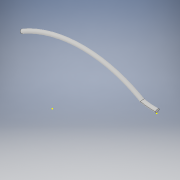
# Autodesk Inventor part: CapBallHolderArmNew
Saved by Autodesk Inventor 2017 (Build 210142000, 142)
## iProperties
Created: 2017-04-24
Part Number: CapBallHolderArmNew
Material: Generic
Document SubType Name: Modeling
Designer: RoboticsUser
Density: 1 g/cm^3
Appearance: Default
Mass: 11.5621 g
Surface Area: 73.9815 cm^2
Volume: 11.5621 cm^3
Author: RoboticsUser
Autodesk Inventor part; units mm, degrees
ref_plane "YZ Plane" through (0, 0, 0) normal (1, 0, 0) x (0, 1, 0)
ref_plane "XZ Plane" through (0, 0, 0) normal (0, 1, 0) x (-1, 0, 0)
ref_plane "XY Plane" through (0, 0, 0) normal (0, 0, 1) x (1, 0, 0)
sketch "Sketch1" plane through (0, 0, 0) normal (0, 0, 1) x (1, 0, 0)
  arc A0 (0, 0) -> (-203.2, 0) centre (-101.6, -175.9764) ccw
  dimension "d0" = 203.2
  dimension "d1" = 203.2
  constraints: 2 point on circle, 1 centre point
  measures "d0" distance of A0.start A0.end
  measures "d1" radius of A0
ref_plane "Work Plane1" through (0, 0, 0) normal (-0.8660254, 0.5, 0) x (-0.5, -0.8660254, 0)
ref_plane "Work Plane2" through (-203.2, 0, 0) normal (-0.8660254, -0.5, 0) x (0.5, -0.8660254, 0)
sketch "Sketch2" plane through (0, 0, 0) normal (-0.8660254, 0.5, 0) x (-0.5, -0.8660254, 0)
  circle A0 centre (0, 0) radius 3.175
  dimension "d2" = 6.35
  constraints: 1 centre point, 1 coincident
  measures "d2" diameter of A0
sketch "Sketch3" plane through (-203.2, 0, 0) normal (-0.8660254, -0.5, 0) x (0.5, -0.8660254, 0)
  circle A0 centre (0, 0) radius 3.175
  point P0 (101.6, 0)
  dimension "d3" = 6.35
  constraints: 1 centre point
  measures "d3" diameter of A0
sweep "Sweep1" add profiles "Sketch3" path "Sketch1"
sketch "Sketch4" plane through (0, 0, 0) normal (-0.8660254, 0.5, 0) x (-0.5, -0.8660254, 0)
  point P0 (0, 0)
sketch "Sketch5" plane through (-203.2, 0, 0) normal (-0.8660254, -0.5, 0) x (0.5, -0.8660254, 0)
  point P0 (101.6, 0)
sketch "Sketch6" plane through (0, 0, 0) normal (0.8660254, -0.5, 0) x (0, 0, 1)
  point P0 (0, 0)
sketch "Sketch7" plane through (0, 0, 0) normal (0, 1, 0) x (-1, 0, 0)
  point P0 (0, 0)
ref_plane "Work Plane3" through (-101.6, -175.9764, 0) normal (0, 0, -1) x (-1, 0, 0)
sketch "Sketch8" plane through (-101.6, -175.9764, 0) normal (0, 0, -1) x (-1, 0, 0)
  arc A0 (-126.913, 173.8763) -> (-101.6, 175.9764) centre (-122.5449, 274.8299) ccw
  dimension "d6" = 25.4
  constraints: 2 point on circle, 1 centre point
  measures "d6" distance of A0.end A0.start
sketch "Sketch9" plane through (0, 0, 0) normal (0.8660254, -0.5, 0) x (0, 0, 1)
  circle A0 centre (0, 0) radius 3.175
  point P0 (0, 0)
  constraints: 1 centre point, 1 coincident
sweep "Sweep2" add profiles "Sketch9" path "Sketch8"
sketch "Sketch10" plane through (25.313, -2.1001, 0) normal (0.9633518, -0.2682411, 0) x (0, 0, -1)
  point P0 (0, -4.7669)
sketch "Sketch11" plane through (-203.2, 0, 0) normal (-0.8660254, -0.5, 0) x (0, 0, -1)
  point P0 (0, 101.6)
body "Solid1"
